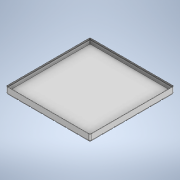
# Autodesk Inventor part: Blank Storage
Saved by Autodesk Inventor 2022.3 (Build 263350000, 350)
## iProperties
Created: 2022-04-21
Part Number: Blank Storage
Material: Generic
Document SubType Name: Modeling
Designer: smiku
Density: 1 g/cm^3
Appearance: Default
Author: smiku
Autodesk Inventor part; units mm, degrees
ref_plane "YZ Plane" through (0, 0, 0) normal (1, 0, 0) x (0, 1, 0)
ref_plane "XZ Plane" through (0, 0, 0) normal (0, 1, 0) x (-1, 0, 0)
sketch "Sketch1" plane through (0, 0, 0) normal (0, 0, 1) x (1, 0, 0)
  line L0 (0, 0) -> (42, 0)
  line L1 (42, 0) -> (42, 42)
  line L2 (42, 42) -> (0, 42)
  line L3 (0, 42) -> (0, 0)
  line L4 (0, 21) -> (42, 21) construction
  line L5 (42, 0) -> (0, 42) construction
  line L6 (0, 14.5) -> (42, 14.5)
  line L7 (0, 27.5) -> (42, 27.5)
  line L8 (27.5, 42) -> (27.5, 0)
  line L9 (14.5, 42) -> (14.5, 0)
  line L10 (14.5, 14.5) -> (0, 0) construction
  circle A0 centre (8, 8) radius 3.25
  circle A1 centre (8, 8) radius 1.5
  circle A2 centre (8, 34) radius 1.5
  circle A3 centre (8, 34) radius 3.25
  circle A4 centre (34, 8) radius 1.5
  circle A5 centre (34, 8) radius 3.25
  circle A6 centre (34, 34) radius 1.5
  circle A7 centre (34, 34) radius 3.25
  point P0 (27.5, 14.5)
  point P1 (27.5, 27.5)
  point P2 (14.5, 27.5)
  dimension "d0" = 42
  dimension "d1" = 42
  dimension "d2" = 13
  dimension "d3" = 8
  dimension "d4" = 3
  dimension "d5" = 6.5
  constraints: 22 end point, 9 point on line, 8 centre point, 6 equal radius, 4 coincident, 4 symmetric about line, 3 perpendicular, 2 horizontal alignment, 2 midpoint, 2 parallel, 2 vertical alignment, 1 horizontal, 1 other
  measures "d0" distance of L1.end L2.end
  measures "d1" distance of L0.end L1.end
  measures "d2" distance between parallel lines of L6 L7
  measures "d3" distance from line of L0 A0.centre
  measures "d4" diameter of A1
  measures "d5" diameter of A0
extrude "Extrusion1" add sketch "Sketch1" along normal blind 5 contours L3 L6 L9 L0 | L9 L6 L8 L0 | L3 L7 L9 L6 | L8 L6 L1 L0 | L9 L7 L8 L6 | L3 L2 L9 L7 | L8 L7 L1 L6 | L9 L2 L8 L7 | L8 L2 L1 L7 | A0 | A1 | A2 | A3 | A4 | A5 | A6 | A7
ref_plane "Work Plane1" through (0, 21, 0) normal (0, -1, 0) x (1, 0, 0)
sketch "Sketch2" plane through (0, 21, 0) normal (0, -1, 0) x (1, 0, 0)
  line L0 (42, 0) -> (0, 0) construction
  line L1 (0, 0) -> (0, 5) construction
  line L2 (42, 5) -> (0, 5) construction
  line L3 (42, 0) -> (42, 5) construction
  line L4 (0, 0) -> (0, 5) projected
  line L5 (0, 5) -> (2.4, 2.6)
  line L6 (2.4, 2.6) -> (2.4, 0.8)
  line L7 (2.4, 0.8) -> (3.2, 0)
  line L8 (42, 0) -> (0, 0) projected
  line L9 (0, 5) -> (-5, 5)
  line L10 (-5, 5) -> (-5, 0)
  line L11 (-5, 0) -> (3.2, 0)
  dimension "d8" = 45
  dimension "d9" = 2.4
  dimension "d10" = 45
  dimension "d11" = 0.8
  constraints: 12 end point, 3 perpendicular, 1 horizontal, 1 parallel, 1 point on line
  measures "d8" angle of L6 L5
  measures "d9" distance between parallel lines of L6 L1
  measures "d10" angle of L11 L7
  measures "d11" horizontal distance of L6.end L7.end
sketch "Sketch3" plane through (0, 0, 5) normal (0, 0, 1) x (1, 0, 0)
  line L0 (4, 0) -> (38, 0)
  line L1 (42, 4) -> (42, 38)
  line L2 (38, 42) -> (4, 42)
  line L3 (0, 38) -> (0, 4)
  arc A0 (4, 42) -> (0, 38) centre (4, 38) ccw
  arc A1 (42, 38) -> (38, 42) centre (38, 38) ccw
  arc A2 (38, 0) -> (42, 4) centre (38, 4) ccw
  arc A3 (0, 4) -> (4, 0) centre (4, 4) ccw
  point P0 (0, 0)
  point P1 (42, 42)
  dimension "d12" = 4
  constraints: 8 end point, 8 point on circle, 8 tangent, 4 centre point, 4 point on line, 3 equal radius, 2 parallel, 1 horizontal, 1 perpendicular
  measures "d12" radius of A0
sweep "Sweep1" cut profiles "Sketch2" path "Sketch3"
extrude "Extrusion2" [suppressed]
feature "FaceDraft1" [suppressed]
extrude "Extrusion3" cut sketch "Sketch1" along normal up to surface (5 mm away) contours A1 | A2 | A4 | A6
extrude "Extrusion4" cut sketch "Sketch1" along normal blind 2.4 contours A0 | A3 | A5 | A7
pattern_linear "Rectangular Pattern1" count 7 spacing 42 along (1, 0, 0) count 7 spacing 42 along (0, 1, 0)
sketch "Sketch4" plane through (0, 0, 5) normal (0, 0, 1) x (1, 0, 0)
  line L0 (4, 0) -> (290, 0)
  line L1 (294, 4) -> (294, 290)
  line L2 (290, 294) -> (4, 294)
  line L3 (0, 290) -> (0, 4)
  arc A0 (0, 4) -> (4, 0) centre (4, 4) ccw
  arc A1 (4, 294) -> (0, 290) centre (4, 290) ccw
  arc A2 (294, 290) -> (290, 294) centre (290, 290) ccw
  arc A3 (290, 0) -> (294, 4) centre (290, 4) ccw
  line L4 (0.25, 4) -> (0.25, 290)
  arc A4 (4, 293.75) -> (0.25, 290) centre (4, 290) ccw
  line L5 (4, 293.75) -> (290, 293.75)
  arc A5 (293.75, 290) -> (290, 293.75) centre (290, 290) ccw
  line L6 (293.75, 290) -> (293.75, 4)
  arc A6 (290, 0.25) -> (293.75, 4) centre (290, 4) ccw
  line L7 (290, 0.25) -> (4, 0.25)
  arc A7 (0.25, 4) -> (4, 0.25) centre (4, 4) ccw
  point P0 (0, 0)
  point P1 (294, 294)
  point P2 (294, 0)
  point P3 (0, 294)
  dimension "d28" = 294
  dimension "d29" = 294
  dimension "d30" = 4
  dimension "d42" = 0.25
  constraints: 16 end point, 16 point on circle, 8 centre point, 8 point on line, 8 tangent, 4 parallel, 3 equal radius, 2 perpendicular, 1 horizontal, 7 other
  measures "d28" distance of point (0, 294) point (294, 294)
  measures "d29" distance of point (294, 0) point (294, 294)
  measures "d30" radius of A0
  measures "d42" distance between parallel lines of L3 L4
extrude "Extrusion5" add sketch "Sketch4" along normal blind 16 contours A0 L3 A1 L2 A2 L1 A3 L0 | L4 A4 L5 A5 L6 A6 L7 A7
sketch "Sketch5" plane through (0, 21, 0) normal (0, -1, 0) x (1, 0, 0)
  line L0 (0, 26) -> (2.4, 23.6)
  line L1 (2.4, 23.6) -> (2.4, 21.8)
  line L2 (2.4, 21.8) -> (3.2, 21)
  line L3 (0, 25.6464) -> (2.15, 23.4964)
  line L4 (2.15, 23.4964) -> (2.15, 21.6964)
  line L5 (2.15, 21.6964) -> (2.8464, 21)
  line L6 (0, 26) -> (0, 21)
  line L7 (0, 21) -> (3.2, 21)
  point P0 (0, 0)
  point P1 (0, 25.6464)
  point P2 (3.0964, 21)
  dimension "d33" = 5
  dimension "d36" = 45
  dimension "d37" = 0.8
  dimension "d38" = 45
  dimension "d39" = 0.25
  dimension "d47" = 2.4
  constraints: 16 end point, 2 point on line, 2 vertical, 1 horizontal alignment, 1 perpendicular, 1 vertical alignment, 2 other
  measures "d33" distance of L6.end L0.start
  measures "d36" angle of L1 L0
  measures "d37" horizontal distance of L1.end L2.end
  measures "d38" angle of L1 L2
  measures "d39" distance between parallel lines of L0 L3
  measures "d47" distance between parallel lines of L1 L6
sweep "Sweep2" add profiles "Sketch5" path "Sketch4" path curves L3 A1 L2 A2 L1 A3 L0 A0 contours L3 L4 L5 L7 L6
extrude "Extrusion6" cut sketch "Sketch4" along normal through all both and the other way through all
fillet "Fillet1" radius 0.6 8 edges at (1.3483, 1.3484, 25.3964) (147, 0.25, 25.3964) (292.6516, 1.3483, 25.3964) (293.75, 147, 25.3964) (292.6514, 292.6519, 25.3964) (147, 293.75, 25.3964) (1.3484, 292.6517, 25.3964) (0.25, 147, 25.3964)
sketch "Sketch6" plane through (0, 0, 21) normal (0, 0, 1) x (1, 0, 0)
  arc A0 (2.8464, 4) -> (4, 2.8464) centre (4, 4) ccw projected
  line L0 (4, 2.8464) -> (290, 2.8464) projected
  arc A1 (290, 2.8464) -> (291.1536, 4) centre (290, 4) ccw projected
  line L1 (291.1536, 4) -> (291.1536, 290) projected
  arc A2 (291.1536, 290) -> (290, 291.1536) centre (290, 290) ccw projected
  line L2 (290, 291.1536) -> (4, 291.1536) projected
  arc A3 (4, 291.1536) -> (2.8464, 290) centre (4, 290) ccw projected
  line L3 (2.8464, 290) -> (2.8464, 4) projected
  point P0 (0, 0)
extrude "Extrusion7" cut sketch "Sketch6" against normal blind 14.8
sketch "Sketch7" plane through (0, 21, 0) normal (0, -1, 0) x (1, 0, 0)
  line L0 (2.8464, 21) -> (2.8464, 6.2) projected
  line L1 (2.8464, 6.2) -> (4, 6.2) projected
  line L2 (2.8464, 6.2) -> (1.45, 6.2)
  line L3 (1.45, 6.2) -> (1.45, 18.4036)
  line L4 (1.45, 18.4036) -> (2.8464, 19.8)
  line L5 (0.25, 4.75) -> (0.25, 23.9479) projected
  point P0 (0, 0)
  dimension "d50" = 45
  dimension "d51" = 1.2
  dimension "d52" = 1.2
  constraints: 6 end point, 1 horizontal, 1 perpendicular, 1 point on line
  measures "d50" angle of L3 L4
  measures "d51" distance between parallel lines of L5 L3
  measures "d52" distance of L0.start L4.end
sweep "Sweep3" cut profiles "Sketch7" path "Sketch4" path curves L3 A1 L2 A2 L1 A3 L0 A0
equation "\"d0\" = slotDimension"
equation "\"d1\" = slotDimension"
equation "\"d2\" = ledStripWidth"
equation "\"d4\" = screwTightDiameter"
equation "\"d5\" = magnetDiameter"
equation "\"d6\" = nestingDepth"
equation "\"d9\" = nestingRimWidth"
equation "\"d12\" = cornerFillet"
equation "\"d15\" = ledSlotHeight"
equation "\"d18\" = ledSlotHeight"
equation "\"d20\" = magnetThiccness"
equation "\"d30\" = cornerFillet"
equation "\"d42\" = nestingClearance"
equation "\"d33\" = nestingDepth"
equation "\"d39\" = nestingClearance"
equation "\"d47\" = nestingRimWidth"
equation "\"d51\" = wallThiccness"
equation "\"d52\" = wallThiccness"
equation "\"d24\" = slotDimension"
equation "\"d27\" = slotDimension"
equation "\"slotsHigh\" = 0.5"
equation "\"slotDimension\" = 42"
equation "\"nestingDepth\" = 5"
equation "\"nestingRimWidth\" = 2.4"
equation "\"cornerFillet\" = 4"
equation "\"ledStripWidth\" = 13"
equation "\"ledSlotHeight\" = 4"
equation "\"screwTightDiameter\" = 3"
equation "\"magnetDiameter\" = 6.5"
equation "\"magnetThiccness\" = 2.4"
equation "\"wallThiccness\" = 1.2"
equation "\"nestingClearance\" = 0.25"
body "Solid1"
